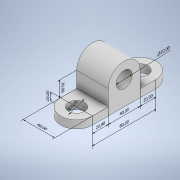
# Autodesk Inventor part: Tarea 1
Saved by Autodesk Inventor 2022 (Build 260153000, 153)
## iProperties
Created: 2024-02-04
Part Number: Tarea 1
Material: Genérico
Document SubType Name: Modeling
Designer: Lourdes Ac Minera
Density: 1 g/cm^3
Appearance: Valor por defecto
Author: Lourdes Ac Minera
Autodesk Inventor part; units mm, degrees
ref_plane "YZ Plane" through (0, 0, 0) normal (1, 0, 0) x (0, 1, 0)
ref_plane "XZ Plane" through (0, 0, 0) normal (0, 1, 0) x (-1, 0, 0)
ref_plane "XY Plane" through (0, 0, 0) normal (0, 0, 1) x (1, 0, 0)
sketch "Boceto1" plane through (0, 0, 0) normal (0, 1, 0) x (-1, 0, 0)
  line L0 (-20, -60) -> (20, -60)
  line L1 (20, -60) -> (20, 60)
  line L2 (20, 60) -> (-20, 60)
  line L3 (-20, 60) -> (-20, -60)
  line L4 (-20, -60) -> (20, 60) construction
  line L5 (20, -60) -> (-20, 60) construction
  line L6 (20, 60) -> (-20, 60)
  line L7 (-20, 60) -> (-20, 20)
  line L8 (-20, 20) -> (20, 20)
  line L9 (20, 20) -> (20, 60)
  line L10 (20, -60) -> (-20, -60)
  line L11 (-20, -60) -> (-20, -20)
  line L12 (-20, -20) -> (20, -20)
  line L13 (20, -20) -> (20, -60)
  circle A0 centre (0, 40) radius 10
  circle A1 centre (0, -40) radius 10
  line L14 (20, 20) -> (-20, 20)
  line L15 (-20, 20) -> (-20, -20)
  line L16 (-20, -20) -> (20, -20)
  line L17 (20, -20) -> (20, 20)
  point P0 (0, 0)
  dimension "d0" = 40
  dimension "d1" = 120
  dimension "d2" = 40
  dimension "d3" = 40
  dimension "d4" = 40
  dimension "d5" = 20
  dimension "d7" = 20
  constraints: 36 end point, 8 parallel, 4 horizontal, 4 perpendicular, 2 centre point, 2 midpoint, 1 point on line
  measures "d0" distance of L2.end L1.end
  measures "d1" distance of L1.end L0.end
  measures "d2" distance of L7.end L6.end
  measures "d3" distance of L11.end L12.end
  measures "d4" distance of L10.end L11.end
  measures "d5" diameter of A0
  measures "d7" diameter of A1
extrude "Extrusión1" add sketch "Boceto1" along normal blind 10
sketch "Boceto2" plane through (0, 10, 0) normal (0, 1, 0) x (1, 0, 0)
  line L0 (-20, -20) -> (20, -20)
  line L1 (20, -20) -> (20, 20)
  line L2 (20, 20) -> (-20, 20)
  line L3 (-20, 20) -> (-20, -20)
  line L4 (-20, -20) -> (20, 20) construction
  line L5 (20, -20) -> (-20, 20) construction
  point P0 (0, 0)
  dimension "d10" = 40
  dimension "d11" = 40
  constraints: 12 end point, 2 midpoint, 2 parallel, 1 horizontal, 1 perpendicular
  measures "d10" distance of L2.end L1.end
  measures "d11" distance of L1.end L0.end
extrude "Extrusión2" add sketch "Boceto2" along normal blind 40
fillet "Empalme de cara1" radius 20 1 edges at (20, 5, 60)
fillet "Empalme de cara2" radius 20 1 edges at (-20, 5, 60)
fillet "Empalme de cara3" radius 20 1 edges at (-20, 5, -60)
fillet "Empalme de cara4" radius 20 1 edges at (20, 5, -60)
sketch "Boceto3" plane through (20, 10, -20) normal (1, 0, 0) x (0, 0, -1)
  line L0 (-60, 0) -> (-40, 0) projected
  circle A0 centre (-20, 20) radius 10
  point P0 (-20, -10)
  dimension "d22" = 20
  constraints: 1 centre point
  measures "d22" diameter of A0
extrude "Extrusión3" cut sketch "Boceto3" against normal blind 40
fillet "Empalme de cara5" radius 20 1 edges at (0, 50, 20)
fillet "Empalme de cara6" radius 20 1 edges at (0, 50, -20)
